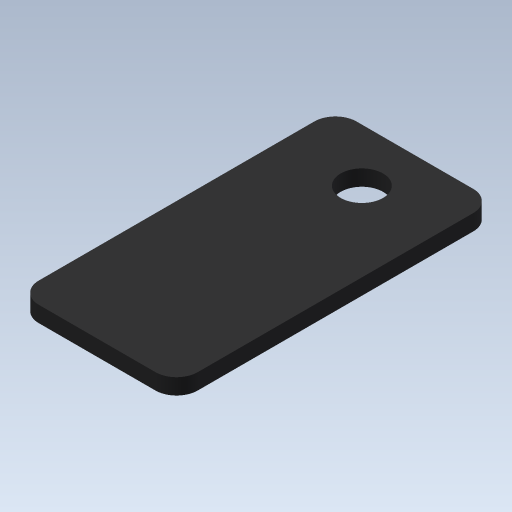
# Autodesk Inventor part: Pump-Motor-CW-Rotation:Valve 101
Saved by Autodesk Inventor 2024.2 (Build 282272000, 272)
## iProperties
Created: 2025-06-16
Document SubType Name: Modeling
Density: 0.93 g/cm^3
Material: Rubber
Mass: 0.60543 g
Surface Area: 10.167 cm^2
Volume: 0.651 cm^3
Appearance: Rubber - Black
Designer: cw
Author: cw
Autodesk Inventor part; units mm, degrees
ref_plane "YZ Plane" through (0, 0, 0) normal (1, 0, 0) x (0, 1, 0)
ref_plane "XZ Plane" through (0, 0, 0) normal (0, 1, 0) x (-1, 0, 0)
ref_plane "XY Plane" through (0, 0, 0) normal (0, 0, 1) x (1, 0, 0)
sketch "Sketch1" plane through (0, 0, 0) normal (0, 0, 1) x (1, 0, 0)
  line L0 (-7.5, 15) -> (7.5, 15)
  line L1 (7.5, 15) -> (7.5, -15)
  line L2 (7.5, -15) -> (-7.5, -15)
  line L3 (-7.5, -15) -> (-7.5, 15)
  circle A0 centre (0, 10) radius 2
  point P0 (0, 0)
  point P1 (-7.5, 0)
  point P2 (0, 15)
  dimension "d0" = 30
  dimension "d1" = 15
  dimension "d5" = 4
  dimension "d7" = 10
  constraints: 8 end point, 2 midpoint, 2 parallel, 2 vertical alignment, 1 centre point, 1 horizontal, 1 horizontal alignment, 1 perpendicular
  measures "d0" distance of L2.end L0.start
  measures "d1" distance of L0.start L0.end
  measures "d5" diameter of A0
  measures "d7" distance of point (0, 0) A0.centre
extrude "Extrusion1" add sketch "Sketch1" along normal blind 1.5
fillet "Fillet1" radius 2 4 edges at (-7.5, 15, 0.75) (7.5, 15, 0.75) (-7.5, -15, 0.75) (7.5, -15, 0.75)
body "Solid1"
